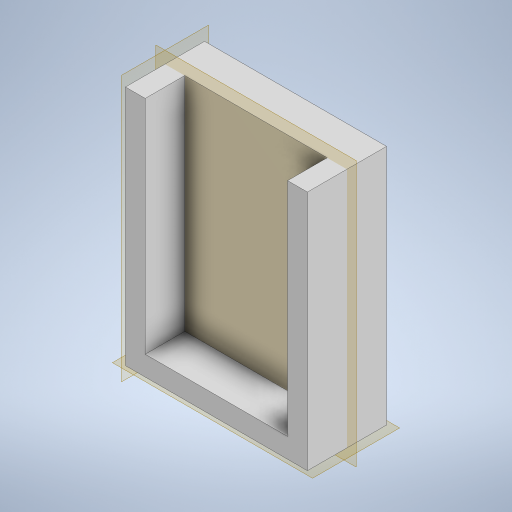
# Autodesk Inventor part: espverkleidung
Saved by Autodesk Inventor 2023 (Build 270158000, 158)
## iProperties
Created: 2025-06-13
Part Number: espverkleidung
Material: Generisch
Document SubType Name: Modeling
Designer: johan
Density: 1 g/cm^3
Appearance: Vorgabe
Author: johan
Autodesk Inventor part; units mm, degrees
sketch "Skizze1" plane through (0, 0, 0) normal (0, 0, 1) x (1, 0, 0)
  line L0 (0, 0) -> (23, 0)
  line L1 (23, 0) -> (23, 30.5)
  line L2 (23, 30.5) -> (0, 30.5)
  line L3 (0, 30.5) -> (0, 0)
  dimension "d0" = 23
  dimension "d1" = 30.5
  constraints: 8 end point, 2 parallel, 1 horizontal, 1 perpendicular
  measures "d0" distance of L2.end L1.end
  measures "d1" distance of L1.end L0.end
extrude "Extrusion1" add sketch "Skizze1" along normal mid plane 10
sketch "Skizze2" plane through (0, 0, 5) normal (0, 0, 1) x (1, 0, 0)
  line L0 (2.5, 28) -> (20.5, 28)
  line L1 (20.5, 28) -> (20.5, 2.5)
  line L2 (20.5, 2.5) -> (2.5, 2.5)
  line L3 (2.5, 2.5) -> (2.5, 28)
  point P0 (0, 0)
  dimension "d4" = 18
  dimension "d5" = 25.5
  constraints: 8 end point, 2 parallel, 1 horizontal, 1 perpendicular
  measures "d4" distance of L1.end L2.end
  measures "d5" distance of L0.end L1.end
extrude "Extrusion2" cut sketch "Skizze2" against normal blind 5
sketch "Skizze3" plane through (0, 30.5, 5) normal (0, 1, 0) x (1, 0, 0)
  line L0 (23, 0) -> (0, 0) projected
  line L1 (2.5, 5) -> (20.5, 5) projected
  line L2 (2.5, 0) -> (20.5, 0)
  line L3 (20.5, 0) -> (20.5, 5)
  line L4 (20.5, 5) -> (2.5, 5)
  line L5 (2.5, 5) -> (2.5, 0)
  point P0 (0, 5)
  dimension "d8" = 18
  dimension "d9" = 5
  constraints: 8 end point, 2 parallel, 1 horizontal, 1 perpendicular, 1 point on line
  measures "d8" distance of L4.end L1.end
  measures "d9" distance of L1.end L2.end
extrude "Extrusion3" cut sketch "Skizze3" against normal blind 5
